Autodesk Fusion 360 part; units mm, degrees
(part 2 of 2)
sketch "Sketch12" plane through (0, 13, 0) normal (0, 1, 0) x (-1, 0, 0) in component "Board"
  line L0 (-150, 7.5) -> (-140, 7.5)
  line L1 (-140, 7.5) -> (-140, -7.5)
  line L2 (-140, -7.5) -> (-150, -7.5)
  line L3 (-150, -7.5) -> (-150, 7.5)
  line L4 (140, -7.5) -> (140, 7.5)
  line L5 (140, 7.5) -> (150, 7.5)
  line L6 (150, 7.5) -> (150, -7.5)
  line L7 (150, -7.5) -> (140, -7.5)
  line L8 (-80, -120) -> (-80, -130)
  line L9 (-80, -130) -> (-70, -130)
  line L10 (-70, -130) -> (-70, -120)
  line L11 (-70, -120) -> (-30, -120)
  line L12 (-30, -120) -> (-30, -130)
  line L13 (-30, -130) -> (-20, -130)
  line L14 (-20, -130) -> (-20, -120)
  line L15 (-20, -120) -> (20, -120)
  line L16 (20, -120) -> (20, -130)
  line L17 (20, -130) -> (30, -130)
  line L18 (30, -130) -> (30, -120)
  line L19 (30, -120) -> (70, -120)
  line L20 (70, -120) -> (70, -130)
  line L21 (70, -130) -> (80, -130)
  line L22 (80, -130) -> (80, -120)
  line L23 (80, -120) -> (120, -120)
  line L24 (120, -120) -> (120, -130)
  line L25 (120, -130) -> (130, -130)
  line L26 (130, -130) -> (130, -120)
  line L27 (130, -120) -> (150, -120)
  line L28 (150, -120) -> (150, -130)
  line L29 (150, -130) -> (160, -130)
  line L30 (160, -130) -> (160, 120)
  line L31 (160, 120) -> (-160, 120)
  line L32 (-160, 120) -> (-160, -130)
  line L33 (-160, -130) -> (-150, -130)
  line L34 (-150, -130) -> (-150, -120)
  line L35 (-150, -120) -> (-130, -120)
  line L36 (-130, -120) -> (-130, -130)
  line L37 (-130, -130) -> (-120, -130)
  line L38 (-120, -130) -> (-120, -120)
  line L39 (-120, -120) -> (-80, -120)
  circle A0 centre (0, 0) radius 12.5
  line L40 (0, 0) -> (-18, 0) construction
  line L41 (-18, 0) -> (-18, 50) construction
  line L42 (-18, 50) -> (-21, 50)
  line L43 (-21, 50) -> (-21, -50)
  line L44 (-21, -50) -> (-18, -50)
  line L45 (-18, -50) -> (-18, 50)
  dimension "d273" = 18
  dimension "d274" = 50
  dimension "d275" = 3
  dimension "d276" = 100
  constraint coincident A0.centre L40.start
  constraint perpendicular L30 L40
  constraint perpendicular L40 L41
  constraint horizontal L42
  constraint vertical L43
  constraint horizontal L44
  constraint vertical L45
  measures "d273" distance of A0.centre L40.end
  measures "d274" distance of L40.end L41.end
  measures "d275" distance of L41.end L42.end
  measures "d276" distance of L41.end L44.end
extrude "Extrude8" add sketch "Sketch12" along normal blind 60 separate body contours L42 L43 L44 L45 makes body 12 in component "Board"
sketch "Sketch13" plane through (0, 13, 0) normal (0, 1, 0) x (-1, 0, 0) in component "Board"
  line L0 (-150, 7.5) -> (-140, 7.5)
  line L1 (-140, 7.5) -> (-140, -7.5)
  line L2 (-140, -7.5) -> (-150, -7.5)
  line L3 (-150, -7.5) -> (-150, 7.5)
  line L4 (140, -7.5) -> (140, 7.5)
  line L5 (140, 7.5) -> (150, 7.5)
  line L6 (150, 7.5) -> (150, -7.5)
  line L7 (150, -7.5) -> (140, -7.5)
  line L8 (-80, -120) -> (-80, -130)
  line L9 (-80, -130) -> (-70, -130)
  line L10 (-70, -130) -> (-70, -120)
  line L11 (-70, -120) -> (-30, -120)
  line L12 (-30, -120) -> (-30, -130)
  line L13 (-30, -130) -> (-20, -130)
  line L14 (-20, -130) -> (-20, -120)
  line L15 (-20, -120) -> (20, -120)
  line L16 (20, -120) -> (20, -130)
  line L17 (20, -130) -> (30, -130)
  line L18 (30, -130) -> (30, -120)
  line L19 (30, -120) -> (70, -120)
  line L20 (70, -120) -> (70, -130)
  line L21 (70, -130) -> (80, -130)
  line L22 (80, -130) -> (80, -120)
  line L23 (80, -120) -> (120, -120)
  line L24 (120, -120) -> (120, -130)
  line L25 (120, -130) -> (130, -130)
  line L26 (130, -130) -> (130, -120)
  line L27 (130, -120) -> (150, -120)
  line L28 (150, -120) -> (150, -130)
  line L29 (150, -130) -> (160, -130)
  line L30 (160, -130) -> (160, 120)
  line L31 (160, 120) -> (-160, 120)
  line L32 (-160, 120) -> (-160, -130)
  line L33 (-160, -130) -> (-150, -130)
  line L34 (-150, -130) -> (-150, -120)
  line L35 (-150, -120) -> (-130, -120)
  line L36 (-130, -120) -> (-130, -130)
  line L37 (-130, -130) -> (-120, -130)
  line L38 (-120, -130) -> (-120, -120)
  line L39 (-120, -120) -> (-80, -120)
  circle A0 centre (0, 0) radius 12.5
  line L40 (0, 0) -> (-18, 0) construction
  line L41 (-18, 0) -> (-18, -50) construction
  line L42 (-18, -50) -> (-21, -50) construction
  line L43 (-21, -50) -> (-21, -30) construction
  line L44 (-21, -30) -> (-18, -30)
  line L45 (-18, -30) -> (-18, -10)
  line L46 (-18, -10) -> (-21, -10)
  line L47 (-21, -10) -> (-21, -30)
  line L48 (-18, 10) -> (-21, 10)
  line L49 (-18, 30) -> (-18, 10)
  line L50 (-21, 10) -> (-21, 30)
  line L51 (-21, 30) -> (-18, 30)
  dimension "d279" = 18
  dimension "d280" = 50
  dimension "d281" = 3
  dimension "d282" = 20
  dimension "d283" = 3
  dimension "d284" = 20
  constraint coincident A0.centre L40.start
  constraint horizontal L40
  constraint perpendicular L40 L41
  constraint perpendicular L41 L42
  constraint perpendicular L42 L43
  constraint horizontal L44
  constraint vertical L45
  constraint horizontal L46
  constraint vertical L47
  constraint symmetric L40 L43.end L50.end
  constraint symmetric L40 L44.end L49.start
  constraint symmetric L40 L45.end L48.start
  constraint symmetric L40 L46.end L48.end
  measures "d279" distance of A0.centre L40.end
  measures "d280" distance of L40.end L41.end
  measures "d281" distance of L41.end L42.end
  measures "d282" distance of L42.end L43.end
  measures "d283" distance of L43.end L44.end
  measures "d284" distance of L43.end L46.end
extrude "Extrude9" cut sketch "Sketch13" against normal blind 5 contours L44 L45 L46 L47 | L48 L49 L50 L51 bodies 4 in component "Board"
sketch "Sketch14" plane through (0, 13, 0) normal (0, -1, 0) x (1, 0, 0) in component "Board"
  line L0 (18, 50) -> (18, -50)
  line L1 (18, -50) -> (21, -50)
  line L2 (21, -50) -> (21, 50)
  line L3 (21, 50) -> (18, 50)
  line L4 (18, -50) -> (18, -30) construction
  line L5 (18, -30) -> (21, -30)
  line L6 (21, -30) -> (21, -10)
  line L7 (21, -10) -> (18, -10)
  line L8 (18, -10) -> (18, -30)
  line L9 (1.75, 0) -> (22.5, 0)
  line L10 (18, 10) -> (18, 30)
  line L11 (21, 10) -> (18, 10)
  line L12 (21, 30) -> (21, 10)
  line L13 (18, 30) -> (21, 30)
  dimension "d287" = 20
  dimension "d288" = 20
  constraint coincident L0.end L1.start
  constraint perpendicular L1 L4
  constraint horizontal L5
  constraint vertical L6
  constraint horizontal L7
  constraint vertical L8
  constraint symmetric L4.end L9 L10.end
  constraint symmetric L5.end L9 L12.start
  constraint symmetric L6.end L9 L11.start
  constraint symmetric L7.end L9 L10.start
  measures "d287" distance of L0.end L4.end
  measures "d288" distance of L4.end L7.end
extrude "Extrude10" add sketch "Sketch14" along normal blind 5 contours L0 L2 L10 L11 L12 L13 | L0 L2 L5 L6 L7 L8 bodies 12 in component "Board"
move_body "Align7" bodies 3 to x (1, 0, 0) y (0, 1, 0) z (0, 0, 1) at (0, -0.25, 0) in component "Slider"
move_body "Align8" bodies 3 to x (1, 0, 0) y (0, 1, 0) z (0, 0, 1) at (0, 0.25, 0) in component "Slider"
sketch "ProjBoard" plane through (0, 8, 0) normal (0, -1, 0) x (1, 0, 0) in component "All"
  line L0 (21, 10) -> (18, 10)
  line L1 (18, 10) -> (18, 30)
  line L2 (18, 30) -> (21, 30)
  line L3 (21, 30) -> (21, 10)
  line L4 (21, -30) -> (18, -30)
  line L5 (18, -30) -> (18, -10)
  line L6 (18, -10) -> (21, -10)
  line L7 (21, -10) -> (21, -30)
  line L8 (140, 7.5) -> (150, 7.5)
  line L9 (150, 7.5) -> (150, -7.5)
  line L10 (150, -7.5) -> (140, -7.5)
  line L11 (140, -7.5) -> (140, 7.5)
  line L12 (-140, 7.5) -> (-140, -7.5)
  line L13 (-140, -7.5) -> (-150, -7.5)
  line L14 (-150, -7.5) -> (-150, 7.5)
  line L15 (-150, 7.5) -> (-140, 7.5)
  circle A0 centre (0, 0) radius 12.5
  line L16 (80, -130) -> (80, -120)
  line L17 (80, -120) -> (120, -120)
  line L18 (120, -120) -> (120, -130)
  line L19 (120, -130) -> (130, -130)
  line L20 (130, -130) -> (130, -120)
  line L21 (130, -120) -> (150, -120)
  line L22 (150, -120) -> (150, -130)
  line L23 (150, -130) -> (160, -130)
  line L24 (160, -130) -> (160, 120)
  line L25 (160, 120) -> (-160, 120)
  line L26 (-160, 120) -> (-160, -130)
  line L27 (-160, -130) -> (-150, -130)
  line L28 (-150, -130) -> (-150, -120)
  line L29 (-150, -120) -> (-130, -120)
  line L30 (-130, -120) -> (-130, -130)
  line L31 (-130, -130) -> (-120, -130)
  line L32 (-120, -130) -> (-120, -120)
  line L33 (-120, -120) -> (-80, -120)
  line L34 (-80, -120) -> (-80, -130)
  line L35 (-80, -130) -> (-70, -130)
  line L36 (-70, -130) -> (-70, -120)
  line L37 (-70, -120) -> (-30, -120)
  line L38 (-30, -120) -> (-30, -130)
  line L39 (-30, -130) -> (-20, -130)
  line L40 (-20, -130) -> (-20, -120)
  line L41 (-20, -120) -> (20, -120)
  line L42 (20, -120) -> (20, -130)
  line L43 (20, -130) -> (30, -130)
  line L44 (30, -130) -> (30, -120)
  line L45 (30, -120) -> (70, -120)
  line L46 (70, -120) -> (70, -130)
  line L47 (70, -130) -> (80, -130)
  line L48 (140, 17.5) -> (140, 7.5)
  line L49 (140, 7.5) -> (150, 7.5)
  line L50 (150, 7.5) -> (150, 17.5)
  line L51 (150, 17.5) -> (140, 17.5)
  line L52 (140, -7.5) -> (140, -17.5)
  line L53 (140, -17.5) -> (150, -17.5)
  line L54 (150, -17.5) -> (150, -7.5)
  line L55 (150, -7.5) -> (140, -7.5)
  line L56 (-140, 7.5) -> (-140, 17.5)
  line L57 (-140, 17.5) -> (-150, 17.5)
  line L58 (-150, 17.5) -> (-150, 7.5)
  line L59 (-150, 7.5) -> (-140, 7.5)
  line L60 (-140, -17.5) -> (-140, -7.5)
  line L61 (-140, -7.5) -> (-150, -7.5)
  line L62 (-150, -7.5) -> (-150, -17.5)
  line L63 (-150, -17.5) -> (-140, -17.5)
sketch "ProjWheel" plane through (0, 0, 0) normal (0, -1, 0) x (1, 0, 0) in component "All"
  circle A0 centre (0, 0) radius 13
  circle A1 centre (0, 100) radius 3
  arc A2 (26.9387, -2.3568) -> (21.6842, -6.0037) centre (26.503, -7.3378) ccw
  line L0 (26.9387, -2.3568) -> (89.1024, -7.7954)
  arc A3 (98.0342, -19.7304) -> (89.1024, -7.7954) centre (88.2308, -17.7574) ccw
  arc A4 (83.2722, -55.3691) -> (98.0342, -19.7304) centre (0, 0) ccw
  arc A5 (68.5171, -57.4927) -> (83.2722, -55.3691) centre (74.945, -49.8322) ccw
  line L1 (68.5171, -57.4927) -> (20.7151, -17.382)
  arc A6 (19.5783, -11.0878) -> (20.7151, -17.382) centre (23.929, -13.5518) ccw
  arc A7 (19.5783, -11.0878) -> (21.6842, -6.0037) centre (0, 0) ccw
  arc A8 (17.382, -20.7151) -> (11.0878, -19.5783) centre (13.5518, -23.929) ccw
  line L2 (17.382, -20.7151) -> (57.4927, -68.5171)
  arc A9 (55.3691, -83.2722) -> (57.4927, -68.5171) centre (49.8322, -74.945) ccw
  arc A10 (19.7304, -98.0342) -> (55.3691, -83.2722) centre (0, 0) ccw
  arc A11 (7.7954, -89.1024) -> (19.7304, -98.0342) centre (17.7574, -88.2308) ccw
  line L3 (7.7954, -89.1024) -> (2.3568, -26.9387)
  arc A12 (6.0037, -21.6842) -> (2.3568, -26.9387) centre (7.3378, -26.503) ccw
  arc A13 (6.0037, -21.6842) -> (11.0878, -19.5783) centre (0, 0) ccw
  arc A14 (2.3568, 26.9387) -> (6.0037, 21.6842) centre (7.3378, 26.503) ccw
  line L4 (2.3568, 26.9387) -> (7.7954, 89.1024)
  arc A15 (19.7304, 98.0342) -> (7.7954, 89.1024) centre (17.7574, 88.2308) ccw
  arc A16 (55.3691, 83.2722) -> (19.7304, 98.0342) centre (0, 0) ccw
  arc A17 (57.4927, 68.5171) -> (55.3691, 83.2722) centre (49.8322, 74.945) ccw
  line L5 (57.4927, 68.5171) -> (17.382, 20.7151)
  arc A18 (11.0878, 19.5783) -> (17.382, 20.7151) centre (13.5518, 23.929) ccw
  arc A19 (11.0878, 19.5783) -> (6.0037, 21.6842) centre (0, 0) ccw
  line L6 (20.7151, 17.382) -> (68.5171, 57.4927)
  arc A20 (83.2722, 55.3691) -> (68.5171, 57.4927) centre (74.945, 49.8322) ccw
  arc A21 (98.0342, 19.7304) -> (83.2722, 55.3691) centre (0, 0) ccw
  arc A22 (89.1024, 7.7954) -> (98.0342, 19.7304) centre (88.2308, 17.7574) ccw
  line L7 (89.1024, 7.7954) -> (26.9387, 2.3568)
  arc A23 (21.6842, 6.0037) -> (26.9387, 2.3568) centre (26.503, 7.3378) ccw
  arc A24 (21.6842, 6.0037) -> (19.5783, 11.0878) centre (0, 0) ccw
  arc A25 (20.7151, 17.382) -> (19.5783, 11.0878) centre (23.929, 13.5518) ccw
  arc A26 (-26.9387, 2.3568) -> (-21.6842, 6.0037) centre (-26.503, 7.3378) ccw
  line L8 (-26.9387, 2.3568) -> (-89.1024, 7.7954)
  arc A27 (-98.0342, 19.7304) -> (-89.1024, 7.7954) centre (-88.2308, 17.7574) ccw
  arc A28 (-83.2722, 55.3691) -> (-98.0342, 19.7304) centre (0, 0) ccw
  arc A29 (-68.5171, 57.4927) -> (-83.2722, 55.3691) centre (-74.945, 49.8322) ccw
  line L9 (-68.5171, 57.4927) -> (-20.7151, 17.382)
  arc A30 (-19.5783, 11.0878) -> (-20.7151, 17.382) centre (-23.929, 13.5518) ccw
  arc A31 (-19.5783, 11.0878) -> (-21.6842, 6.0037) centre (0, 0) ccw
  line L10 (-2.3568, -26.9387) -> (-7.7954, -89.1024)
  arc A32 (-19.7304, -98.0342) -> (-7.7954, -89.1024) centre (-17.7574, -88.2308) ccw
  arc A33 (-55.3691, -83.2722) -> (-19.7304, -98.0342) centre (0, 0) ccw
  arc A34 (-57.4927, -68.5171) -> (-55.3691, -83.2722) centre (-49.8322, -74.945) ccw
  line L11 (-57.4927, -68.5171) -> (-17.382, -20.7151)
  arc A35 (-11.0878, -19.5783) -> (-17.382, -20.7151) centre (-13.5518, -23.929) ccw
  arc A36 (-11.0878, -19.5783) -> (-6.0037, -21.6842) centre (0, 0) ccw
  arc A37 (-2.3568, -26.9387) -> (-6.0037, -21.6842) centre (-7.3378, -26.503) ccw
  arc A38 (-6.0037, 21.6842) -> (-2.3568, 26.9387) centre (-7.3378, 26.503) ccw
  arc A39 (-6.0037, 21.6842) -> (-11.0878, 19.5783) centre (0, 0) ccw
  arc A40 (-17.382, 20.7151) -> (-11.0878, 19.5783) centre (-13.5518, 23.929) ccw
  line L12 (-17.382, 20.7151) -> (-57.4927, 68.5171)
  arc A41 (-55.3691, 83.2722) -> (-57.4927, 68.5171) centre (-49.8322, 74.945) ccw
  arc A42 (-19.7304, 98.0342) -> (-55.3691, 83.2722) centre (0, 0) ccw
  arc A43 (-7.7954, 89.1024) -> (-19.7304, 98.0342) centre (-17.7574, 88.2308) ccw
  line L13 (-7.7954, 89.1024) -> (-2.3568, 26.9387)
  line L14 (-20.7151, -17.382) -> (-68.5171, -57.4927)
  arc A44 (-83.2722, -55.3691) -> (-68.5171, -57.4927) centre (-74.945, -49.8322) ccw
  arc A45 (-98.0342, -19.7304) -> (-83.2722, -55.3691) centre (0, 0) ccw
  arc A46 (-89.1024, -7.7954) -> (-98.0342, -19.7304) centre (-88.2308, -17.7574) ccw
  line L15 (-89.1024, -7.7954) -> (-26.9387, -2.3568)
  arc A47 (-21.6842, -6.0037) -> (-26.9387, -2.3568) centre (-26.503, -7.3378) ccw
  arc A48 (-21.6842, -6.0037) -> (-19.5783, -11.0878) centre (0, 0) ccw
  arc A49 (-20.7151, -17.382) -> (-19.5783, -11.0878) centre (-23.929, -13.5518) ccw
  circle A50 centre (0, 0) radius 110
sketch "ProjBackLayer" plane through (0, 5, 0) normal (0, -1, 0) x (1, 0, 0) in component "All"
  circle A0 centre (4.75, -8.2272) radius 1.5
  circle A1 centre (-4.75, 8.2272) radius 1.5
  circle A2 centre (9.5, 0) radius 1.5
  circle A3 centre (-4.75, -8.2272) radius 1.5
  circle A4 centre (-9.5, 0) radius 1.5
  circle A5 centre (4.75, 8.2272) radius 1.5
  circle A6 centre (0, 0) radius 110
sketch "ProjSlider" plane through (0, -5, 0) normal (0, -1, 0) x (1, 0, 0) in component "All"
  arc A0 (-3.25, -100) -> (3.25, -100) centre (0, -100) ccw
  line L0 (-3.25, -100) -> (-3.25, 100)
  arc A1 (3.25, 100) -> (-3.25, 100) centre (0, 100) ccw
  line L1 (3.25, 100) -> (3.25, -100)
  arc A2 (13.25, 100) -> (-13.25, 100) centre (0, 100) ccw
  line L2 (-13.25, 100) -> (-13.25, 7.5)
  line L3 (-13.25, 7.5) -> (-268.25, 7.5)
  line L4 (-268.25, 7.5) -> (-268.25, -7.5)
  line L5 (-268.25, -7.5) -> (-13.25, -7.5)
  line L6 (-13.25, -7.5) -> (-13.25, -100)
  arc A3 (-13.25, -100) -> (13.25, -100) centre (0, -100) ccw
  line L7 (13.25, -100) -> (13.25, -7.5)
  line L8 (13.25, -7.5) -> (268.25, -7.5)
  line L9 (268.25, -7.5) -> (268.25, 7.5)
  line L10 (268.25, 7.5) -> (13.25, 7.5)
  line L11 (13.25, 7.5) -> (13.25, 100)
sketch "ProjHolder4Slider" plane through (-150, 0, 0) normal (-1, 0, 0) x (0, -1, 0) in component "All"
  arc A0 (12, 7.5) -> (2, 17.5) centre (2, 7.5) ccw
  line L0 (2, 17.5) -> (-8, 17.5)
  line L1 (-8, 17.5) -> (-8, 7.5)
  line L2 (-8, 7.5) -> (-13, 7.5)
  line L3 (-13, 7.5) -> (-13, -7.5)
  line L4 (-13, -7.5) -> (-8, -7.5)
  line L5 (-8, -7.5) -> (-8, -17.5)
  line L6 (-8, -17.5) -> (2, -17.5)
  arc A1 (2, -17.5) -> (12, -7.5) centre (2, -7.5) ccw
  line L7 (12, -7.5) -> (12, 7.5)
  line L8 (-0.25, 7.75) -> (5.25, 7.75)
  line L9 (5.25, 7.75) -> (5.25, -7.75)
  line L10 (5.25, -7.75) -> (-0.25, -7.75)
  line L11 (-0.25, -7.75) -> (-0.25, 7.75)
sketch "ProjHolder4Motor" plane through (18, 0, 0) normal (-1, 0, 0) x (0, -1, 0) in component "All"
  line L0 (-13, -50) -> (-13, -30)
  line L1 (-13, -30) -> (-8, -30)
  line L2 (-8, -30) -> (-8, -10)
  line L3 (-8, -10) -> (-13, -10)
  line L4 (-13, -10) -> (-13, 10)
  line L5 (-13, 10) -> (-8, 10)
  line L6 (-8, 10) -> (-8, 30)
  line L7 (-8, 30) -> (-13, 30)
  line L8 (-13, 30) -> (-13, 50)
  line L9 (-13, 50) -> (-73, 50)
  line L10 (-73, 50) -> (-73, -50)
  line L11 (-73, -50) -> (-13, -50)
sketch "ProjBase" plane through (0, 0, -120) normal (0, 0, 1) x (-1, 0, 0) in component "All"
  line L0 (-150, -43) -> (150, -43)
  line L1 (150, -43) -> (150, 5)
  line L2 (150, 5) -> (-150, 5)
  line L3 (-150, 5) -> (-150, -43)
  line L4 (-130, -13) -> (-130, -8)
  line L5 (-130, -8) -> (-120, -8)
  line L6 (-120, -8) -> (-120, -13)
  line L7 (-120, -13) -> (-130, -13)
  line L8 (130, -8) -> (130, -13)
  line L9 (130, -13) -> (120, -13)
  line L10 (120, -13) -> (120, -8)
  line L11 (120, -8) -> (130, -8)
  line L12 (-80, -13) -> (-80, -8)
  line L13 (-80, -8) -> (-70, -8)
  line L14 (-70, -8) -> (-70, -13)
  line L15 (-70, -13) -> (-80, -13)
  line L16 (80, -13) -> (70, -13)
  line L17 (70, -13) -> (70, -8)
  line L18 (70, -8) -> (80, -8)
  line L19 (80, -8) -> (80, -13)
  line L20 (-30, -13) -> (-30, -8)
  line L21 (-30, -8) -> (-20, -8)
  line L22 (-20, -8) -> (-20, -13)
  line L23 (-20, -13) -> (-30, -13)
  line L24 (30, -13) -> (20, -13)
  line L25 (20, -13) -> (20, -8)
  line L26 (20, -8) -> (30, -8)
  line L27 (30, -8) -> (30, -13)
sketch "ProjHangerBase" plane through (13.25, 0, 0) normal (1, 0, 0) x (0, 1, 0) in component "All"
  line L0 (-15.1, -90) -> (-15.1, -98)
  line L1 (-15.1, -98) -> (-18.2, -98)
  line L2 (-18.2, -98) -> (-18.2, -90)
  line L3 (-18.2, -90) -> (-20.2, -90)
  line L4 (-20.2, -90) -> (-20.2, -100)
  line L5 (-20.2, -100) -> (-5, -100)
  line L6 (-5, -100) -> (-5, -90)
  line L7 (-5, -90) -> (-15.1, -90)
  circle A0 centre (-10.05, -95) radius 3.05
sketch "ProjHangerPc1" plane through (13.25, 0, 0) normal (-1, 0, 0) x (0, -1, 0) in component "All"
  circle A0 centre (10.05, -95) radius 3
  circle A1 centre (10.05, -95) radius 4.5
  circle A2 centre (10.05, -95) radius 3
  circle A3 centre (10.05, -95) radius 4.5
sketch "ProjHangerPc2" plane through (0, -18.1, 0) normal (0, -1, 0) x (1, 0, 0) in component "All"
  circle A0 centre (0, -94) radius 3
  line L0 (13.25, -98) -> (13.25, -90)
  line L1 (13.25, -90) -> (-13.25, -90)
  line L2 (-13.25, -90) -> (-13.25, -98)
  line L3 (-13.25, -98) -> (13.25, -98)
sketch "ProjSlider2" plane through (0, -5, 0) normal (0, -1, 0) x (1, 0, 0) in component "All"
  arc A0 (-3.25, -100) -> (3.25, -100) centre (0, -100) ccw
  line L0 (-3.25, -100) -> (-3.25, 100)
  arc A1 (3.25, 100) -> (-3.25, 100) centre (0, 100) ccw
  line L1 (3.25, 100) -> (3.25, -100)
  arc A2 (13.25, 100) -> (-13.25, 100) centre (0, 100) ccw
  line L2 (-13.25, 100) -> (-13.25, 7.5)
  line L3 (-13.25, 7.5) -> (-268.25, 7.5)
  line L4 (-268.25, 7.5) -> (-268.25, -7.5)
  line L5 (-268.25, -7.5) -> (-13.25, -7.5)
  line L6 (-13.25, -7.5) -> (-13.25, -100)
  arc A3 (-13.25, -100) -> (13.25, -100) centre (0, -100) ccw
  line L7 (13.25, -100) -> (13.25, -7.5)
  line L8 (13.25, -7.5) -> (268.25, -7.5)
  line L9 (268.25, -7.5) -> (268.25, 7.5)
  line L10 (268.25, 7.5) -> (13.25, 7.5)
  line L11 (13.25, 7.5) -> (13.25, 100)
  line L12 (3.25, -90) -> (3.25, -100)
  line L13 (3.25, -100) -> (13.25, -100)
  line L14 (13.25, -100) -> (13.25, -90)
  line L15 (13.25, -90) -> (3.25, -90)
  line L16 (-13.25, -90) -> (-13.25, -100)
  line L17 (-13.25, -100) -> (-3.25, -100)
  line L18 (-3.25, -100) -> (-3.25, -90)
  line L19 (-3.25, -90) -> (-13.25, -90)
sketch "ProjBackLayer2" plane through (0, 5, 0) normal (0, -1, 0) x (1, 0, 0) in component "All"
  circle A0 centre (4.75, -8.2272) radius 1.5
  circle A1 centre (-4.75, 8.2272) radius 1.5
  circle A2 centre (9.5, 0) radius 1.5
  circle A3 centre (-4.75, -8.2272) radius 1.5
  circle A4 centre (-9.5, 0) radius 1.5
  circle A5 centre (4.75, 8.2272) radius 1.5
  circle A6 centre (0, 0) radius 110
  circle A7 centre (0, 0) radius 13
  circle A8 centre (0, 0) radius 110
component "All" placed x (1, 0, 0) y (0, 1, 0) z (0, 0, 1) at (0, 0, 0)
component "Wheel" placed x (1, 0, 0) y (0, 1, 0) z (0, 0, 1) at (0, 0, 0) in component "All"
component "BackWheel" placed x (1, 0, 0) y (0, 1, 0) z (0, 0, 1) at (0, 5, 0) in component "All"
component "Slider" placed x (1, 0, 0) y (0, 1, 0) z (0, 0, 1) at (-1.75, 0, -0.25) in component "All"
component "Board" placed x (1, 0, 0) y (0, 1, 0) z (0, 0, 1) at (0, 0, 0) in component "All"
component "Base" placed x (1, 0, 0) y (0, 1, 0) z (0, 0, 1) at (0, 0, 0) in component "All"
component "HangerBase" placed x (1, 0, 0) y (0, 1, 0) z (0, 0, 1) at (0, 0, 0) in component "All"
component "HangerSideways" placed x (1, 0, 0) y (0, 1, 0) z (0, 0, 1) at (0, 0, 0) in component "All"
component "HangerOutin" placed x (1, 0, 0) y (0, 1, 0) z (0, 0, 1) at (0, 0, 0) in component "All"
